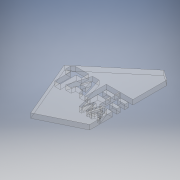
# Autodesk Inventor part: Tage logo 2,0
Saved by Autodesk Inventor 2018 (Build 220112000, 112)
## iProperties
Created: 2018-10-30
Part Number: Tage logo 2,0
Material: Generic
Document SubType Name: Modeling
Designer: Otis PC
Density: 1 g/cm^3
Appearance: Polycarbonate - Clear
Author: Otis PC
Autodesk Inventor part; units mm, degrees
ref_plane "YZ Plane" through (0, 0, 0) normal (1, 0, 0) x (0, 1, 0)
ref_plane "XZ Plane" through (0, 0, 0) normal (0, 1, 0) x (-1, 0, 0)
ref_plane "XY Plane" through (0, 0, 0) normal (0, 0, 1) x (1, 0, 0)
sketch "Sketch1" plane through (0, 0, 0) normal (0, 0, 1) x (1, 0, 0)
  line L0 (18.5838, -6.189) -> (18.5838, 42.8381)
  line L1 (18.5838, 42.8381) -> (12.2763, 47.2547)
  line L2 (12.2763, 47.2547) -> (-22.1957, 18.3292)
  line L3 (-22.1957, 18.3292) -> (-6.5665, -18.491)
  line L4 (18.5838, -6.189) -> (-6.5665, -18.491)
  point P0 (0, 0)
  dimension "d69" = 125
  dimension "d70" = 116.065
  dimension "d71" = 50
  dimension "d72" = 23
  dimension "d73" = 18.5838
  dimension "d74" = 45.7502
  dimension "d75" = 13.7251
  dimension "d76" = 28.3081
  dimension "d77" = 13.2695
  constraints: 10 end point, 1 vertical
  measures "d69" angle of L1 L0
  measures "d70" angle of L0 L4
  measures "d71" angle of L0 L2
  measures "d72" angle of L0 L3
  measures "d73" distance from line of point (0, 0) L0
  measures "d74" distance from line of point (0, 0) L1
  measures "d75" distance from line of point (0, 0) L4
  measures "d76" distance from line of point (0, 0) L2
  measures "d77" distance from line of point (0, 0) L3
sketch "Sketch2" plane through (0, 0, 0) normal (0, 0, 1) x (1, 0, 0)
  line L0 (-9.5924, 21.2326) -> (-17.8048, 21.2326)
  line L1 (-19.5924, 19.7326) -> (-19.5924, 16.7326)
  line L2 (-9.5924, 16.7326) -> (-9.5924, 21.2326)
  line L3 (-16.447, 6.6055) -> (-12.947, 6.6055)
  line L4 (-12.947, 6.6055) -> (-12.947, 16.7326)
  line L5 (-12.947, 21.2326) -> (-16.447, 21.2326)
  line L6 (-16.447, 16.7326) -> (-16.447, 6.6055)
  line L7 (-19.5924, 16.7326) -> (-16.447, 16.7326)
  line L8 (-12.947, 16.7326) -> (-9.5924, 16.7326)
  line L9 (-6.9955, 10.5461) -> (-2.6955, 10.5461)
  line L10 (-3.2476, 13.1461) -> (-6.4988, 13.1461)
  line L11 (-6.9955, 10.5461) -> (-7.5373, 8.1055)
  line L12 (-2.6955, 10.5461) -> (-2.1538, 8.1055)
  line L13 (1.1842, 8.1055) -> (-2.9398, 21.2326)
  line L14 (-10.8158, 8.1055) -> (-6.9955, 21.2326)
  line L15 (-4.8455, 18.2326) -> (-6.4988, 13.1461)
  line L16 (-4.8455, 18.2326) -> (-3.2476, 13.1461)
  line L17 (-2.9398, 21.2326) -> (-6.9955, 21.2326)
  line L18 (-9.5924, 21.2326) -> (-10.8158, 21.2326)
  line L19 (-10.8158, 8.1055) -> (-7.5373, 8.1055)
  line L20 (-2.1538, 8.1055) -> (1.1842, 8.1055)
  line L21 (1.7053, 8.1055) -> (4.7053, 8.1055)
  line L22 (4.7053, 21.2326) -> (1.7053, 21.2326)
  line L23 (1.7053, 21.2326) -> (1.7053, 8.1055)
  line L24 (4.7053, 21.2326) -> (10.0053, 21.2326)
  line L25 (10.0053, 21.2326) -> (10.0053, 18.2326)
  line L26 (10.0053, 18.2326) -> (4.7053, 18.2326)
  line L27 (4.7053, 12.8401) -> (9.7053, 12.8401)
  line L28 (9.7053, 12.8401) -> (9.7053, 15.8401)
  line L29 (9.7053, 15.8401) -> (4.7053, 15.8401)
  line L30 (4.7053, 8.1055) -> (4.7053, 12.8401)
  line L31 (4.7053, 18.2326) -> (4.7053, 15.8401)
  line L32 (10.6316, 8.1055) -> (13.9316, 8.1055)
  line L33 (13.9316, 21.2326) -> (10.6316, 21.2326)
  line L34 (10.6316, 21.2326) -> (10.6316, 8.1055)
  line L35 (10.6316, 21.2326) -> (18.5838, 21.2326)
  line L36 (18.5838, 21.2326) -> (18.5838, 18.2326)
  line L37 (18.5838, 18.2326) -> (13.9316, 18.2326)
  line L38 (10.6316, 18.2326) -> (10.6316, 21.2326)
  line L39 (10.6316, 8.1055) -> (18.5838, 8.1055)
  line L40 (18.5838, 8.1055) -> (18.5838, 11.1055)
  line L41 (18.5838, 11.1055) -> (13.9316, 11.1055)
  line L42 (10.6316, 11.1055) -> (10.6316, 8.1055)
  line L43 (18.5838, 13.169) -> (13.9316, 13.169)
  line L44 (10.6316, 13.169) -> (10.6316, 16.169)
  line L45 (13.9316, 16.169) -> (18.5838, 16.169)
  line L46 (18.5838, 16.169) -> (18.5838, 13.169)
  line L47 (13.9316, 11.1055) -> (13.9316, 13.169)
  line L48 (13.9316, 16.169) -> (13.9316, 18.2326)
  line L49 (4.7101, 7.4818) -> (6.2371, 1.7828)
  line L50 (4.7101, 7.4818) -> (10.6101, 7.4818) construction
  line L51 (6.2371, 1.7828) -> (7.5531, 7.4818)
  line L52 (6.6393, 0.4313) -> (8.1922, 6.2269)
  line L53 (6.6393, 0.4313) -> (12.6393, 0.4313) construction
  line L54 (8.1922, 6.2269) -> (9.6357, 0.4313)
  line L55 (8.9116, 7.4818) -> (10.1897, 1.7237)
  line L56 (10.1897, 1.7237) -> (11.7321, 7.4799)
  line L57 (5.2852, 0.4313) -> (6.6393, 0.4313)
  line L58 (12.7416, 7.4799) -> (10.6898, 0.4313)
  line L59 (9.6357, 0.4313) -> (10.6898, 0.4313)
  line L60 (8.9116, 7.4818) -> (7.5531, 7.4818)
  line L61 (11.7321, 7.4799) -> (12.7416, 7.4799)
  line L62 (3.6715, 7.4818) -> (4.7101, 7.4818)
  line L63 (3.6715, 7.4818) -> (5.2852, 0.4313)
  line L64 (18.0899, 0.4313) -> (18.0899, 1.2146)
  line L65 (15.6901, 7.4818) -> (14.2447, 7.4818)
  line L66 (14.2447, 7.4818) -> (15.6901, 7.4818)
  line L67 (18.0899, 1.2146) -> (18.0899, 0.4313)
  line L68 (18.0899, 0.4313) -> (16.9444, 0.4313)
  line L69 (14.2447, 7.4818) -> (12.0899, 1.2146)
  line L70 (15.6901, 7.4818) -> (18.0899, 1.2146)
  line L71 (14.2447, 3.278) -> (15.8544, 3.278)
  line L72 (13.7758, 1.9143) -> (16.3765, 1.9143)
  line L73 (13.2659, 0.4313) -> (13.7758, 1.9143)
  line L74 (14.2447, 3.278) -> (15.0062, 5.4929)
  line L75 (15.0062, 5.4929) -> (15.8544, 3.278)
  line L76 (16.3765, 1.9143) -> (16.9444, 0.4313)
  line L77 (12.0899, 0.4313) -> (13.2659, 0.4313)
  line L78 (16.9444, 0.4313) -> (18.0899, 0.4313)
  line L79 (12.0899, 1.2146) -> (12.0899, 0.4313)
  line L80 (-19.5924, 19.7326) -> (-17.8048, 21.2326)
  line L81 (-19.5924, 19.7326) -> (-17.2589, 19.7326) construction
  point P0 (0, 0)
  dimension "d39" = 3
  dimension "d41" = 12
  dimension "d44" = 2.5
  dimension "d45" = 2.5
  dimension "d46" = 3
  dimension "d47" = 5.3
  dimension "d48" = 5
  dimension "d49" = 3
  dimension "d50" = 3.3
  dimension "d51" = 3
  dimension "d52" = 3
  dimension "d55" = 5.9
  dimension "d56" = 75
  dimension "d57" = 6
  dimension "d58" = 75
  dimension "d62" = 40
  constraints: 164 end point, 35 parallel, 19 horizontal, 14 perpendicular, 4 point on line, 3 equal length, 2 collinear
  measures "d39" distance of L1.end L1.start
  measures "d41" distance of L14.start L13.start
  measures "d44" distance of L9.start L11.end
  measures "d45" distance of L9.end L12.end
  measures "d46" distance of L22.end L22.start
  measures "d47" distance of L25.end L26.end
  measures "d48" distance of L29.end L28.end
  measures "d49" distance of L28.end L27.end
  measures "d50" distance of L33.end L33.start
  measures "d51" distance of L40.end L39.end
  measures "d52" distance of L44.start L44.end
  measures "d55" distance of L49.start L49.end
  measures "d56" angle of L49 L50
  measures "d57" distance of L52.start L52.end
  measures "d58" angle of L53 L52
  measures "d62" angle of L81 L80
extrude "Extrusion1" add sketch "Sketch1" against normal blind 3
extrude "Extrusion2" cut sketch "Sketch2" against normal blind 3
body "Solid1"
